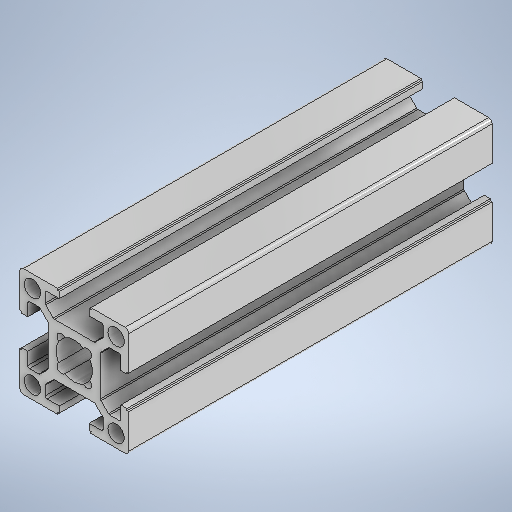
# Autodesk Inventor part: Perfil 30×30 4 rasgos_001
Saved by Autodesk Inventor 2026 (Build 300175000, 175)
## iProperties
Created: 2025-04-05
Part Number: Perfil 30×30 4 rasgos_001
Material: Aluminum 6061
Document SubType Name: Modeling
Designer: Tony Dias
Density: 2.7 g/cm^3
Appearance: Aluminum - Polished
Author: Tony Dias
Autodesk Inventor part; units mm, degrees
sketch "Sketch1" plane through (0, 0, 0) normal (0, 0, 1) x (1, 0, 0)
  circle A0 centre (0, 0) radius 5 construction
  line L0 (-15, 15) -> (0, 0) construction
  circle A1 centre (-11.5, 11.5) radius 2.25
  line L1 (-7.2, 7.2) -> (0, 7.2) construction
  line L2 (-7.2, 7.2) -> (-7.2, 0) construction
  line L3 (-8, 9.5556) -> (-5.6444, 7.2)
  line L4 (-9.5556, 8) -> (-7.2, 5.6444)
  line L5 (-15, 15) -> (-15, 4.1) construction
  line L6 (-15, 4.1) -> (-12.8, 4.1) construction
  line L7 (-12.8, 8) -> (-9.5556, 8)
  line L8 (-12.8, 8) -> (-12.8, 4.1)
  line L9 (-15, 15) -> (-4.1, 15) construction
  line L10 (-4.1, 15) -> (-4.1, 12.8) construction
  line L11 (-4.1, 12.8) -> (-8, 12.8)
  line L12 (-8, 12.8) -> (-8, 9.5556)
  line L13 (-7.2, 5.6444) -> (-7.2, 0)
  circle A2 centre (-3.5355, 3.5355) radius 1.25 construction
  circle A3 centre (-3.5355, -3.5355) radius 1.25 construction
  circle A4 centre (3.5355, -3.5355) radius 1.25 construction
  circle A5 centre (3.5355, 3.5355) radius 1.25 construction
  line L14 (-7.2, 0) -> (-5, 0)
  line L15 (-5.6444, 7.2) -> (0, 7.2)
  line L16 (0, 7.2) -> (0, 5)
  line L17 (-15, 4.1) -> (-14.5, 4.1) construction
  line L18 (-14.5, 4.1) -> (-14.5, 4.6)
  line L19 (-14.5, 4.6) -> (-15, 4.6)
  line L20 (-15, 4.6) -> (-15, 4.1) construction
  line L21 (-4.1, 15) -> (-4.6, 15) construction
  line L22 (-4.6, 15) -> (-4.6, 14.5)
  line L23 (-4.6, 14.5) -> (-4.1, 14.5)
  line L24 (-4.1, 14.5) -> (-4.1, 15) construction
  line L25 (-4.1, 14.5) -> (-4.1, 12.8)
  line L26 (-15, 15) -> (-15, 4.6)
  line L27 (-14.5, 4.1) -> (-12.8, 4.1)
  line L28 (-15, 15) -> (-4.6, 15)
  arc A6 (-4.302, 2.5481) -> (-5, 0) centre (0, 0) ccw
  arc A7 (-2.5481, 4.302) -> (-4.302, 2.5481) centre (-3.5355, 3.5355) ccw
  arc A8 (0, 5) -> (-2.5481, 4.302) centre (0, 0) ccw
  dimension "d0" = 10
  dimension "d2" = 15
  dimension "d3" = 15
  dimension "d4" = 4.5
  dimension "d5" = 11.5
  dimension "d6" = 11.5
  dimension "d7" = 2.2
  dimension "d9" = 1.1
  dimension "d10" = 4.1
  dimension "d11" = 2.2
  dimension "d13" = 1.25
  dimension "d14" = 4.1
  dimension "d15" = 2.5
  dimension "d18" = 360
  dimension "d20" = 0.5
  constraints: 58 end point, 13 point on circle, 11 horizontal, 9 centre point, 9 vertical, 7 coincident, 6 equal length, 5 parallel, 4 point on line, 3 concentric, 2 perpendicular, 1 horizontal alignment, 1 vertical alignment, 10 other
  measures "d0" diameter of A0
  measures "d2" horizontal distance of point (0, 0) L0.start
  measures "d3" horizontal distance of point (0, 0) L0.start
  measures "d4" diameter of A1
  measures "d5" horizontal distance of point (0, 0) A1.centre
  measures "d6" horizontal distance of point (0, 0) A1.centre
  measures "d7" distance edge to line of A0 L1
  measures "d9" distance between parallel lines of L0 L3
  measures "d10" vertical distance of point (0, 0) L5.end
  measures "d11" distance of L5.end L6.end
  measures "d13" distance edge to line of A1 L7
  measures "d14" horizontal distance of point (0, 0) L9.end
  measures "d15" diameter of A2
  measures "d20" distance of L18.end L19.end
extrude "Extrusion1" add sketch "Sketch1" along normal mid plane 100
mirror "Mirror1" about plane through (0, 0, 0) normal (1, 0, 0) of "Extrusion1"
mirror "Mirror2" about plane through (0, 0, 0) normal (0, 1, 0) of "Extrusion1", "Mirror1"
fillet "Fillet1" radius 1 4 edges at (-15, 15, 0) (15, 15, 0) (15, -15, 0) (-15, -15, 0)
fillet "Fillet2" radius 0.5 24 edges at (-9.5556, -8, 0) (9.5556, -8, 0) (7.2, -5.6444, 0) (-5.6444, 7.2, 0) (-8, 9.5556, 0) (5.6444, 7.2, 0) (-12.8, -8, 0) (-8, -12.8, 0) (-7.2, 5.6444, 0) (-9.5556, 8, 0) (-12.8, 8, 0) (-8, 12.8, 0) (7.2, 5.6444, 0) (9.5556, 8, 0) (-5.6444, -7.2, 0) (-8, -9.5556, 0) (5.6444, -7.2, 0) (8, -9.5556, 0) (8, -12.8, 0) (12.8, -8, 0) (8, 9.5556, 0) (-7.2, -5.6444, 0) (12.8, 8, 0) (8, 12.8, 0)
equation "\"d2\" = d3"
equation "\"d11\" = d7"
equation "\"d14\" = d10"
body "Solid1"
